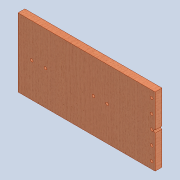
# Autodesk Inventor part: 0005-10-024
Saved by Autodesk Inventor 2020 (Build 240168000, 168)
## iProperties
Created: 2020-12-18
Part Number: 0005-10-024
Material: Generic
Document SubType Name: Modeling
Designer: Iulian Bors
Density: 1 g/cm^3
Appearance: White Oak - Natural Medium Gloss
Author: Iulian Bors
Subject: 024
Autodesk Inventor part; units mm, degrees
ref_plane "YZ Plane" through (0, 0, 0) normal (1, 0, 0) x (0, 1, 0)
ref_plane "XZ Plane" through (0, 0, 0) normal (0, 1, 0) x (-1, 0, 0)
ref_plane "XY Plane" through (0, 0, 0) normal (0, 0, 1) x (1, 0, 0)
sketch "Sketch1" plane through (0, 0, 0) normal (0, 0, 1) x (1, 0, 0)
  line L0 (-200, 100) -> (200, 100)
  line L1 (200, 100) -> (200, -100)
  line L2 (200, -100) -> (-200, -100)
  line L3 (-200, -100) -> (-200, 100)
  point P0 (0, 0)
  point P1 (0, 100)
  point P2 (-200, 0)
  dimension "d0" = 400
  dimension "d1" = 200
  constraints: 8 end point, 2 midpoint, 2 parallel, 1 horizontal, 1 horizontal alignment, 1 perpendicular, 1 vertical alignment
  measures "d0" distance of L0.start L0.end
  measures "d1" distance of L2.end L0.start
extrude "Extrusion1" add sketch "Sketch1" along normal mid plane 20
sketch "Sketch10" plane through (0, 0, 10) normal (0, 0, 1) x (1, 0, 0)
  line L0 (-200, 100) -> (-200, -100) projected
  point P0 (0, 0)
  point P1 (-160, 0)
  dimension "d53" = 40
  constraints: 1 horizontal alignment
  measures "d53" distance from line of point (-160, 0) L0
hole "Hole1" at (-160, 0, 10) direction (0, 0, -1) diameter 8 end through all
pattern_linear "Rectangular Pattern1" count 2 spacing 40 along (1, 0, 0) count 2 spacing 180 along (1, 0, 0) of "Hole1"
sketch "Sketch11" plane through (0, 0, 10) normal (0, 0, 1) x (1, 0, 0)
  line L0 (200, -100) -> (200, 100) projected
  point P0 (0, 0)
  point P1 (190, 0)
  point P2 (200, 0)
  dimension "d57" = 10
  constraints: 1 horizontal alignment, 1 midpoint
  measures "d57" distance from line of L0 point (190, 0)
hole "Hole2" at (190, 0, 10) direction (0, 0, -1) diameter 8 end through all
pattern_linear "Rectangular Pattern2" count 5 spacing 40 along (0, 1, 0) of "Hole2" first direction both ways yes
body "Solid1"
